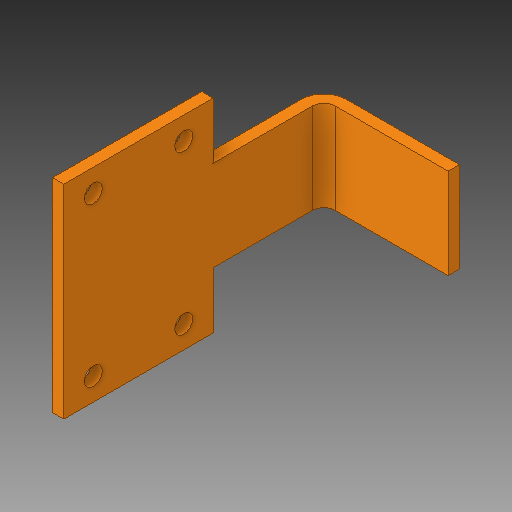
# Autodesk Inventor part: motor mount
Saved by Autodesk Inventor 2017 SP1 (Build 210196100, 196)
## iProperties
Created: 2018-01-26
Part Number: motor mount
Material: Aluminum 6061
Document SubType Name: Modeling
Designer: Ben
Density: 2.7 g/cm^3
Appearance: Orange
Mass: 34.4634 g
Surface Area: 92.987 cm^2
Volume: 12.7642 cm^3
Author: Ben
Autodesk Inventor part; units mm, degrees
ref_plane "YZ Plane" through (0, 0, 0) normal (1, 0, 0) x (0, 1, 0)
ref_plane "XZ Plane" through (0, 0, 0) normal (0, 1, 0) x (-1, 0, 0)
ref_plane "XY Plane" through (0, 0, 0) normal (0, 0, 1) x (1, 0, 0)
sketch "Sketch1" plane through (0, 0, 0) normal (0, 1, 0) x (-1, 0, 0)
  line L0 (-38.1, 0) -> (0, 0)
  line L1 (0, 0) -> (0, 76.2)
  line L2 (0, 76.2) -> (-3.175, 76.2)
  line L3 (-38.1, 0) -> (-38.1, 3.175)
  line L4 (-38.1, 3.175) -> (-3.175, 3.175)
  line L5 (-3.175, 3.175) -> (-3.175, 76.2)
  dimension "d0" = 38.1
  dimension "d1" = 76.2
  dimension "d2" = 3.175
  constraints: 12 end point, 5 perpendicular, 1 horizontal, 1 vertical
  measures "d0" distance of L0.start L0.end
  measures "d1" distance of L0.end L1.end
  measures "d2" distance of L1.end L2.end
extrude "Extrusion1" add sketch "Sketch1" along normal blind 57.15
sketch "Sketch2" plane through (38.1, 0, 3.175) normal (1, 0, 0) x (0, 0, -1)
  line L0 (3.175, 57.15) -> (-31.115, 57.15)
  line L1 (-31.115, 57.15) -> (-31.115, 41.275)
  line L2 (-31.115, 41.275) -> (3.175, 41.275)
  line L3 (3.175, 41.275) -> (3.175, 57.15)
  line L4 (3.175, 0) -> (-31.115, 0)
  line L5 (-31.115, 0) -> (-31.115, 15.875)
  line L6 (-31.115, 15.875) -> (3.175, 15.875)
  line L7 (3.175, 15.875) -> (3.175, 0)
  line L8 (-64.77, 50.8) -> (-39.37, 50.8) construction
  line L9 (-39.37, 50.8) -> (-39.37, 6.35) construction
  line L10 (-39.37, 6.35) -> (-64.77, 6.35) construction
  line L11 (-64.77, 6.35) -> (-64.77, 50.8) construction
  line L12 (-52.07, 50.8) -> (-52.07, 57.15) construction
  line L13 (-52.07, 6.35) -> (-52.07, 0) construction
  line L14 (-73.025, 57.15) -> (0, 57.15) construction
  line L15 (0, 0) -> (-73.025, 0) construction
  circle A0 centre (-39.37, 50.8) radius 2.54
  circle A1 centre (-64.77, 50.8) radius 2.54
  circle A2 centre (-39.37, 6.35) radius 2.54
  circle A3 centre (-64.77, 6.35) radius 2.54
  line L16 (-73.025, 0) -> (-73.025, 57.15) construction
  line L17 (-39.37, 50.8) -> (-31.115, 50.8) construction
  line L18 (-64.77, 50.8) -> (-73.025, 50.8) construction
  dimension "d5" = 25.4
  dimension "d6" = 44.45
  dimension "d8" = 5.08
  dimension "d9" = 25.4
  dimension "d10" = 41.91
  constraints: 32 end point, 6 parallel, 6 point on line, 4 centre point, 4 coincident, 4 perpendicular, 3 collinear, 3 equal radius, 3 horizontal, 2 midpoint, 2 vertical
  measures "d5" distance between parallel lines of L6 L2
  measures "d6" distance of L10.end L8.start
  measures "d8" diameter of A0
  measures "d9" distance of L8.start L8.end
  measures "d10" distance between parallel lines of L16 L1
extrude "Extrusion2" cut sketch "Sketch2" against normal through all
fillet "Fillet1" radius 3.175 1 edges at (3.175, 28.575, 3.175)
fillet "Fillet1" radius 6.35 1 edges at (0, 28.575, 0)
body "Solid1"
